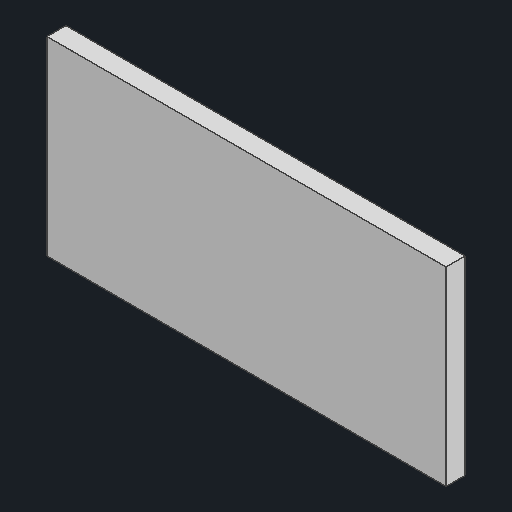
# Autodesk Inventor part: base3
Saved by Autodesk Inventor 2026 (Build 300175000, 175)
## iProperties
Created: 2026-08-17
Part Number: base3
Material: Generic
Document SubType Name: Modeling
Designer: imcle
Density: 1 g/cm^3
Appearance: Default
Author: imcle
Autodesk Inventor part; units mm, degrees
ref_plane "YZ Plane" through (0, 0, 0) normal (1, 0, 0) x (0, 1, 0)
ref_plane "XZ Plane" through (0, 0, 0) normal (0, 1, 0) x (-1, 0, 0)
ref_plane "XY Plane" through (0, 0, 0) normal (0, 0, 1) x (1, 0, 0)
sketch "Sketch2" plane through (0, 0, 0) normal (0, 0, 1) x (1, 0, 0)
  line L0 (0, 0) -> (126, 0)
  line L1 (126, 0) -> (126, 60)
  line L2 (126, 60) -> (0, 60)
  line L3 (0, 60) -> (0, 0)
  dimension "d1" = 126
  dimension "d2" = 60
  constraints: 8 end point, 2 parallel, 1 horizontal, 1 perpendicular
  measures "d1" distance of L2.end L1.end
  measures "d2" distance of L1.end L0.end
extrude "Extrusion1" add sketch "Sketch2" along normal blind 6
sketch "Sketch3" plane through (126, 0, 0) normal (1, 0, 0) x (0, 0, -1)
  line L0 (0, 0) -> (-6, 0) projected
  line L1 (-3, 0) -> (-3, 11)
  circle A0 centre (-3, 11) radius 2
  dimension "d5" = 11
  dimension "d6" = 4
  constraints: 2 end point, 1 centre point, 1 coincident, 1 midpoint, 1 vertical
  measures "d5" distance of L1.start L1.end
  measures "d6" diameter of A0
extrude "Extrusion2" add sketch "Sketch3" against normal blind 5.5
body "Solid2"
